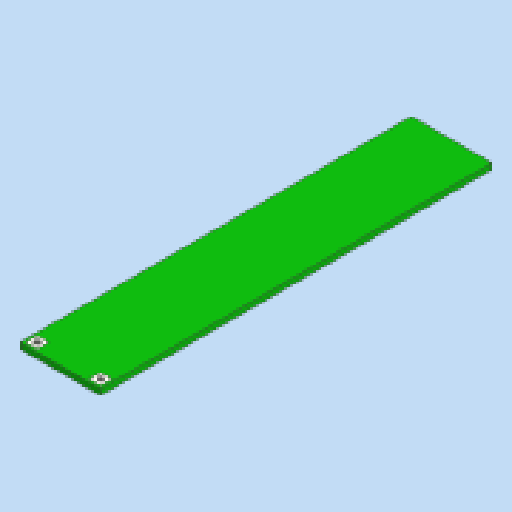
# Autodesk Inventor part: MCU_PCB
Saved by Autodesk Inventor 2024 (Build 280153000, 153)
## iProperties
Created: 2025-02-15
Part Number: MCU_PCB
Material: Generic
Document SubType Name: Modeling
Designer: XxPan
Density: 1 g/cm^3
Appearance: Default
Author: XxPan
Autodesk Inventor part; units mm, degrees
ref_plane "YZ Plane" through (0, 0, 0) normal (1, 0, 0) x (0, 1, 0)
ref_plane "XZ Plane" through (0, 0, 0) normal (0, 1, 0) x (-1, 0, 0)
ref_plane "XY Plane" through (0, 0, 0) normal (0, 0, 1) x (1, 0, 0)
sketch "Sketch1" plane through (0, 0, 0) normal (0, 1, 0) x (-1, 0, 0)
  line L0 (7, 34) -> (-7, 34)
  line L1 (-7, 34) -> (-7, -34)
  line L2 (-7, -34) -> (7, -34)
  line L3 (7, -34) -> (7, 34)
  line L4 (9.8, 0) -> (-9.8, 0) construction
  line L5 (0, -47.6) -> (0, 47.6) construction
  point P0 (0, 0)
  point P1 (7, 0)
  point P2 (0, 34)
  dimension "d0" = 14
  dimension "d1" = 68
  constraints: 8 end point, 2 midpoint, 2 parallel, 2 point on line, 1 horizontal, 1 perpendicular
  measures "d0" distance of L2.end L1.end
  measures "d1" distance of L2.end L0.start
extrude "Extrusion1" add sketch "Sketch1" along normal mid plane 1
sketch "Sketch3" plane through (0, 0.5, 0) normal (0, 1, 0) x (1, 0, 0)
  circle A0 centre (5.5, -32.5) radius 0.5
  circle A1 centre (-5.5, -32.5) radius 0.5
  line L0 (-7, -34) -> (7, -34) projected
  line L1 (7, -34) -> (7, 34) projected
  line L2 (-7, 34) -> (-7, -34) projected
  point P0 (0, 0)
  dimension "d8" = 1
  dimension "d9" = 1
  dimension "d10" = 1.5
  dimension "d11" = 1.5
  dimension "d12" = 1.5
  constraints: 2 centre point, 1 horizontal alignment
  measures "d8" diameter of A0
  measures "d9" diameter of A1
  measures "d10" distance from line of L0 A0.centre
  measures "d11" distance from line of L1 A0.centre
  measures "d12" distance from line of L2 A1.centre
extrude "Extrusion3" cut sketch "Sketch3" against normal through all
sketch "Sketch4" plane through (0, 0.5, 0) normal (0, 1, 0) x (1, 0, 0)
  line L0 (6.5, -31.5) -> (4.5, -31.5)
  line L1 (4.5, -31.5) -> (4.5, -33.5)
  line L2 (4.5, -33.5) -> (6.5, -33.5)
  line L3 (6.5, -33.5) -> (6.5, -31.5)
  line L4 (-4.5, -31.5) -> (-6.5, -31.5)
  line L5 (-6.5, -31.5) -> (-6.5, -33.5)
  line L6 (-6.5, -33.5) -> (-4.5, -33.5)
  line L7 (-4.5, -33.5) -> (-4.5, -31.5)
  circle A0 centre (5.5, -32.5) radius 0.5 construction
  circle A1 centre (-5.5, -32.5) radius 0.5 construction
  point P0 (0, 0)
  point P1 (4.5, -32.5)
  point P2 (-5.5, -31.5)
  point P3 (5.5, -31.5)
  dimension "d15" = 2
  dimension "d16" = 2
  dimension "d17" = 2
  dimension "d18" = 2
  constraints: 16 end point, 4 parallel, 3 midpoint, 2 horizontal, 2 perpendicular, 2 vertical alignment, 1 horizontal alignment, 1 point on line
  measures "d15" distance of L2.end L1.end
  measures "d16" distance of L1.end L0.end
  measures "d17" distance of L6.end L5.end
  measures "d18" distance of L5.end L4.end
surface extrude "ExtrusionSrf1" sketch "Sketch4" against normal through all shown yes curves L7 L4 L5 L6
surface extrude "ExtrusionSrf2" sketch "Sketch4" against normal through all shown yes curves L1 L2 L3 L0
split_face "Split1"
split_face "Split2"
body "Solid1"
body "Srf1"
body "Srf2"
